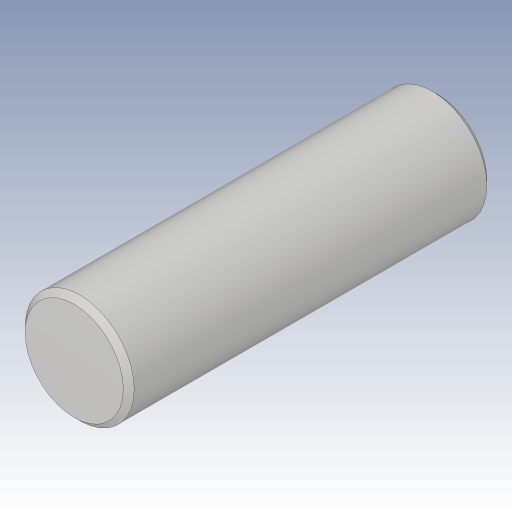
# Autodesk Inventor part: Nummer?
Saved by Autodesk Inventor 2023.3 (Build 273359000, 359)
## iProperties
Company: HTBLA Kaindorf
RuleStatus: InUse
Created: 2023-08-12
Part Number: Nummer?
Project: Fiberprinter-Hotend
Material: Kupfer
Description: Bauteilname?
Document SubType Name: Modeling
Designer: Konstrukteur?
Mass: 5.04079 g
Surface Area: 4.2668 cm^2
Volume: 0.563847 cm^3
Density: 8.94 g/cm^3
Appearance: Satin
AfterDocNew0: iProperties-Editor_aufrufen
Author: nicob
Keywords: Schuljahr?
Autodesk Inventor part; units mm, degrees
ref_plane "YZ Plane" through (0, 0, 0) normal (1, 0, 0) x (0, 1, 0)
ref_plane "XZ Plane" through (0, 0, 0) normal (0, 1, 0) x (-1, 0, 0)
ref_plane "XY Plane" through (0, 0, 0) normal (0, 0, 1) x (1, 0, 0)
sketch "Skizze3" plane through (0, 0, 0) normal (1, 0, 0) x (0, 1, 0)
  circle A0 centre (0, 0) radius 3
  dimension "d4" = 6
  constraints: 1 centre point, 1 coincident
  measures "d4" diameter of A0
extrude "Extrusion3" add sketch "Skizze3" along normal blind 20
chamfer "Fase1" distance 0.3 angle 45 2 edges at (0, -3, 0) (20, -3, 0)
